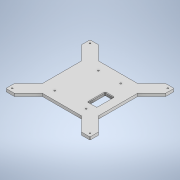
# Autodesk Inventor part: agv_nano_base
Saved by Autodesk Inventor 2021.3 (Build 253353010, 353A)
## iProperties
Created: 2021-04-20
Part Number: agv_nano_base
Material: Generic
Document SubType Name: Modeling
Designer: jesse
Density: 1 g/cm^3
Appearance: Default
Author: jesse
Autodesk Inventor part; units mm, degrees
ref_plane "YZ Plane" through (0, 0, 0) normal (1, 0, 0) x (0, 1, 0)
ref_plane "XZ Plane" through (0, 0, 0) normal (0, 1, 0) x (-1, 0, 0)
ref_plane "XY Plane" through (0, 0, 0) normal (0, 0, 1) x (1, 0, 0)
sketch "Sketch2" plane through (0, 0, 0) normal (0, 1, 0) x (-1, 0, 0)
  line L0 (67.9954, 72.8645) -> (-82.0046, 72.8645)
  line L1 (-82.0046, 72.8645) -> (-82.0046, -77.1355)
  line L2 (-82.0046, -77.1355) -> (67.9954, -77.1355)
  line L3 (67.9954, -77.1355) -> (67.9954, 72.8645)
  circle A0 centre (62.4954, 67.3645) radius 1.3
  line L4 (67.9954, -2.1355) -> (-82.0046, -2.1355)
  line L5 (-7.0046, 72.8645) -> (-7.0046, -77.1355)
  circle A1 centre (62.4954, -71.6355) radius 1.3
  circle A2 centre (-76.5046, 67.3645) radius 1.3
  circle A3 centre (-76.5046, -71.6355) radius 1.3
  point P0 (0, 0)
  dimension "d0" = 150
  dimension "d1" = 150
  dimension "d2" = 5.5
  dimension "d3" = 5.5
  dimension "d43" = 2.6
  constraints: 12 end point, 4 centre point, 4 midpoint, 3 symmetric about line, 2 parallel, 1 horizontal, 1 perpendicular, 3 other
  measures "d0" distance of L2.end L0.start
  measures "d1" distance of L1.end L2.end
  measures "d2" distance from line of L3 A0.centre
  measures "d3" distance from line of A0.centre L0
  measures "d43" diameter of A3
extrude "Extrusion1" add sketch "Sketch2" along normal blind 5
sketch "Sketch4" plane through (0, 5, 0) normal (0, 1, 0) x (1, 0, 0)
  line L0 (-12.9954, 37.1355) -> (27.0046, 37.1355)
  line L1 (27.0046, 37.1355) -> (35.0046, -32.8645)
  line L2 (35.0046, -32.8645) -> (-20.9954, -32.8645)
  line L3 (-20.9954, -32.8645) -> (-12.9954, 37.1355)
  line L4 (7.0046, 37.1355) -> (7.0046, -32.8645)
  line L5 (82.0046, -72.8645) -> (82.0046, 77.1355) projected
  line L6 (-16.9954, 2.1355) -> (31.0046, 2.1355)
  line L7 (82.0046, 77.1355) -> (-67.9954, 77.1355) projected
  circle A0 centre (-12.9954, 37.1355) radius 1.3
  circle A1 centre (27.0046, 37.1355) radius 1.3
  circle A2 centre (35.0046, -32.8645) radius 1.3
  circle A3 centre (-20.9954, -32.8645) radius 1.3
  line L8 (26.5046, 9.6355) -> (41.5046, 9.6355)
  line L9 (41.5046, 9.6355) -> (41.5046, -20.3645)
  line L10 (41.5046, -20.3645) -> (26.5046, -20.3645)
  line L11 (26.5046, -20.3645) -> (26.5046, 9.6355)
  line L12 (26.5046, -5.3645) -> (41.5046, -5.3645)
  line L13 (34.0046, 9.6355) -> (34.0046, -20.3645)
  point P0 (0, 0)
  dimension "d17" = 40
  dimension "d18" = 56
  dimension "d19" = 75
  dimension "d20" = 75
  dimension "d21" = 2.6
  dimension "d22" = 2.6
  dimension "d23" = 2.6
  dimension "d24" = 2.6
  dimension "d45" = 70
  dimension "d51" = 15
  dimension "d52" = 30
  dimension "d53" = 27.5
  dimension "d54" = 1
  constraints: 24 end point, 8 midpoint, 4 centre point, 4 coincident, 3 parallel, 2 horizontal, 2 perpendicular
  measures "d17" distance of L0.start L0.end
  measures "d18" distance of L1.end L2.end
  measures "d19" distance between parallel lines of L5 L4
  measures "d20" distance between parallel lines of L7 L6
  measures "d21" diameter of A0
  measures "d22" diameter of A1
  measures "d23" diameter of A2
  measures "d24" diameter of A3
  measures "d45" distance of L4.start L4.end
  measures "d51" distance of L8.start L8.end
  measures "d52" distance of L8.end L9.end
  measures "d53" distance from line of L1.end L12
  measures "d54" distance from line of L1.end L13
extrude "Extrusion6" cut sketch "Sketch4" against normal through all contours L3 A0 L0 | L0 A0 L3 | A1 L1 L0 | L0 L1 A1 | A3 L2 L3 | L3 L2 A3 | L11 L8 L1 L6 | L6 L1 L12 L11 | L8 L13 L12 L1 | A2 L1 L2 | L2 L1 A2 | L12 L1 L10 L11 | L8 L9 L12 L13 | L12 L13 L10 L1 | L12 L9 L10 L13
fillet "Fillet5" radius 1 12 edges at (26.5046, 5, 5.3645) (34.0046, 5, -9.6355) (41.5046, 5, 5.3645) (34.0046, 5, 20.3645) (82.0046, 2.5, 72.8645) (82.0046, 2.5, -77.1355) (-67.9954, 2.5, 72.8645) (-67.9954, 2.5, -77.1355) (41.5046, 2.5, -9.6355) (26.5046, 2.5, -9.6355) (26.5046, 2.5, 20.3645) (41.5046, 2.5, 20.3645)
sketch "Sketch8" plane through (0, 5, 0) normal (0, 1, 0) x (1, 0, 0)
  line L0 (-67.9954, 76.1355) -> (-67.9954, -71.8645) projected
  line L1 (-67.9954, 62.1355) -> (-42.9954, 37.1355)
  line L2 (-42.9954, 37.1355) -> (-42.9954, -32.8645)
  line L3 (-42.9954, -32.8645) -> (-67.9954, -57.8645)
  line L4 (81.0046, 77.1355) -> (-66.9954, 77.1355) projected
  line L5 (7.0046, 77.1355) -> (7.0046, -72.8645)
  line L6 (-66.9954, -72.8645) -> (81.0046, -72.8645) projected
  line L7 (82.0046, 62.1355) -> (57.0046, 37.1355)
  line L8 (57.0046, 37.1355) -> (57.0046, -32.8645)
  line L9 (57.0046, -32.8645) -> (82.0046, -57.8645)
  line L10 (-52.9954, 77.1355) -> (-27.9954, 52.1355)
  line L11 (-27.9954, 52.1355) -> (42.0046, 52.1355)
  line L12 (42.0046, 52.1355) -> (67.0046, 77.1355)
  line L13 (-52.9954, -72.8645) -> (-27.9954, -47.8645)
  line L14 (-27.9954, -47.8645) -> (42.0046, -47.8645)
  line L15 (42.0046, -47.8645) -> (67.0046, -72.8645)
  line L16 (82.0046, -71.8645) -> (82.0046, 76.1355) projected
  point P0 (0, 0)
  dimension "d56" = 25
  dimension "d57" = 15
  dimension "d58" = 15
  dimension "d59" = 25
  dimension "d60" = 25
  dimension "d61" = 15
  dimension "d62" = 15
  dimension "d63" = 15
  dimension "d64" = 25
  dimension "d65" = 25
  constraints: 26 end point, 6 point on line, 4 symmetric about line, 3 parallel, 2 midpoint, 2 perpendicular, 1 horizontal
  measures "d56" distance between parallel lines of L2 L0
  measures "d57" distance from line of L4 L1.start
  measures "d58" distance from line of L6 L3.end
  measures "d59" horizontal distance of L1.start L1.end
  measures "d60" horizontal distance of L3.end L2.end
  measures "d61" distance from line of L0 L13.start
  measures "d62" distance from line of L15.end L16
  measures "d63" distance from line of L16 L12.end
  measures "d64" distance from line of L6 L13.end
  measures "d65" distance from line of L6 L14.end
extrude "Extrusion7" cut sketch "Sketch8" against normal through all
equation "\"d1\" = d0"
equation "\"d22\" = d21"
equation "\"d23\" = d21"
equation "\"d24\" = d21"
body "Solid1"
